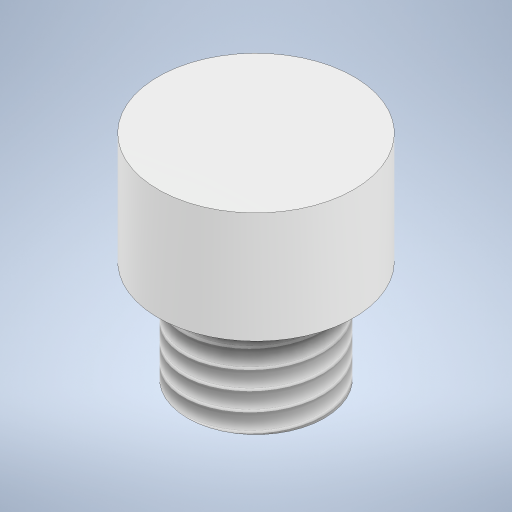
# Autodesk Inventor part: Acople con rosca
Saved by Autodesk Inventor 2024 (Build 280153000, 153)
## iProperties
Created: 2022-09-01
Part Number: Acople con rosca
Material: PVC, no plastificado
Document SubType Name: Modeling
Designer: Usuario
Density: 1.29 g/cm^3
Appearance: Suave - Blanco
Mass: 9.53929 g
Surface Area: 51.1122 cm^2
Volume: 7.3948 cm^3
Author: Usuario
Autodesk Inventor part; units mm, degrees
ref_plane "YZ Plane" through (0, 0, 0) normal (1, 0, 0) x (0, 1, 0)
ref_plane "XZ Plane" through (0, 0, 0) normal (0, 1, 0) x (-1, 0, 0)
sketch "Boceto1" plane through (0, 0, 0) normal (0, 1, 0) x (-1, 0, 0)
  circle A0 centre (0, 0) radius 9
  circle A1 centre (0, 0) radius 13.325
  dimension "d0" = 18
  dimension "d1" = 26.65
  constraints: 2 centre point, 2 coincident
  measures "d0" diameter of A0
  measures "d1" diameter of A1
extrude "Extrusión1" add sketch "Boceto1" against normal blind 23.6
ref_plane "Plano de trabajo2" through (0, -18.5, 0) normal (0, 1, 0) x (1, 0, 0)
sketch "Boceto4" plane through (0, -18.5, 0) normal (0, 1, 0) x (1, 0, 0)
  circle A0 centre (0, 0) radius 6.8
  dimension "d18" = 13.6
  constraints: 1 centre point, 1 coincident
  measures "d18" diameter of A0
extrude "Extrusión4" add sketch "Boceto4" against normal blind 18.97
sketch "Boceto5" plane through (0, 0, 0) normal (0, 1, 0) x (1, 0, 0)
  circle A0 centre (0, 0) radius 10.7
  constraints: 1 centre point, 1 coincident
extrude "Extrusión5" cut sketch "Boceto5" against normal blind 18.97
sketch "Boceto6" plane through (0, -37.47, 0) normal (0, -1, 0) x (1, 0, 0)
  circle A0 centre (0, 0) radius 6.7
  circle A1 centre (0, 0) radius 9.3
  dimension "d25" = 13.4
  dimension "d26" = 18.6
  constraints: 2 centre point, 2 coincident
  measures "d25" diameter of A0
  measures "d26" diameter of A1
extrude "Extrusión6" add sketch "Boceto6" against normal blind 18.97
sketch "Boceto7" plane through (0, -37.47, 0) normal (0, -1, 0) x (1, 0, 0)
  circle A0 centre (0, 0) radius 8.5
  dimension "d29" = 17
  constraints: 1 centre point, 1 coincident
  measures "d29" diameter of A0
extrude "Extrusión7" cut sketch "Boceto7" against normal blind 18.97
thread "Rosca2" size "M20x2.5" class "6g" standard "ANSI Metric M Profile" full length
sketch "Boceto9" plane through (0, -37.47, 0) normal (0, -1, 0) x (1, 0, 0)
  circle A0 centre (0, 0) radius 9.3
  constraints: 1 centre point, 1 coincident
extrude "Extrusión8" cut sketch "Boceto9" along normal blind 8.47
sketch "Boceto10" plane through (0, -23.6, 0) normal (0, -1, 0) x (1, 0, 0)
  circle A0 centre (0, 0) radius 10.7
  constraints: 1 centre point, 1 coincident
extrude "Extrusión9" add sketch "Boceto10" against normal blind 1
sketch "Boceto11" plane through (0, -23.6, 0) normal (0, -1, 0) x (1, 0, 0)
  circle A0 centre (0, 0) radius 8.5
  constraints: 1 centre point, 1 coincident
extrude "Extrusión10" cut sketch "Boceto11" against normal blind 53.22
sketch "Boceto12" plane through (0, 0, 0) normal (0, 1, 0) x (1, 0, 0)
  circle A0 centre (0, 0) radius 8.5 projected
  circle A1 centre (0, 0) radius 10.7
  circle A2 centre (0, 0) radius 9.3 projected
  circle A3 centre (0, 0) radius 13.88
  constraints: 2 centre point, 2 coincident
extrude "Extrusión11" cut sketch "Boceto12" against normal blind 8.47 contours A3
sketch "Boceto13" plane through (0, -8.47, 0) normal (0, 1, 0) x (1, 0, 0)
  circle A0 centre (0, 0) radius 10.7 projected
  circle A1 centre (0, 0) radius 10.7
  constraints: 1 centre point, 1 coincident, 1 concentric
extrude "Extrusión12" add sketch "Boceto13" against normal up to surface (15.13 mm away)
sketch "Boceto14" plane through (0, -37.47, 0) normal (0, -1, 0) x (1, 0, 0)
  circle A0 centre (0, 0) radius 8.5 projected
  circle A1 centre (0, 0) radius 8.5
  constraints: 1 centre point, 1 coincident, 1 concentric
extrude "Extrusión13" add sketch "Boceto14" against normal up to surface (13.87 mm away)
sketch "Boceto15" plane through (0, -37.47, 0) normal (0, -1, 0) x (1, 0, 0)
  circle A0 centre (0, 0) radius 9.3 projected
  circle A1 centre (0, 0) radius 9.3
  dimension "d46" = 18.6
  constraints: 1 centre point, 1 coincident, 1 concentric
  measures "d46" diameter of A0
